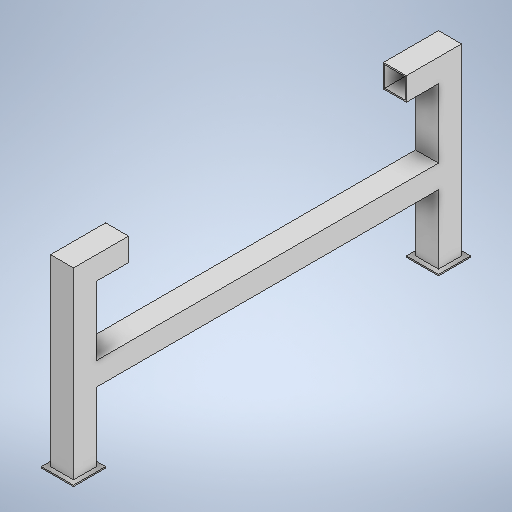
# Autodesk Inventor part: Soporte_altura
Saved by Autodesk Inventor 2025.2 (Build 292293000, 293)
## iProperties
Created: 2025-11-06
Part Number: Soporte_altura
Material: Genérico
Document SubType Name: Modeling
Designer: Dax
Density: 1 g/cm^3
Appearance: Valor por defecto
Author: Dax
Autodesk Inventor part; units mm, degrees
ref_plane "YZ Plane" through (0, 0, 0) normal (1, 0, 0) x (0, 1, 0)
ref_plane "XZ Plane" through (0, 0, 0) normal (0, 1, 0) x (-1, 0, 0)
ref_plane "XY Plane" through (0, 0, 0) normal (0, 0, 1) x (1, 0, 0)
sketch "Boceto1" plane through (0, 0, 0) normal (0, 0, 1) x (1, 0, 0)
  line L0 (-15.875, -15.875) -> (15.875, -15.875)
  line L1 (15.875, -15.875) -> (15.875, 15.875)
  line L2 (15.875, 15.875) -> (-15.875, 15.875)
  line L3 (-15.875, 15.875) -> (-15.875, -15.875)
  line L4 (-15.875, -15.875) -> (15.875, 15.875) construction
  line L5 (15.875, -15.875) -> (-15.875, 15.875) construction
  line L6 (-17.875, 17.875) -> (17.875, 17.875)
  line L7 (17.875, 17.875) -> (17.875, -17.875)
  line L8 (17.875, -17.875) -> (-17.875, -17.875)
  line L9 (-17.875, -17.875) -> (-17.875, 17.875)
  point P0 (0, 0)
  dimension "d0" = 31.75
  dimension "d1" = 31.75
  dimension "d2" = 2
  constraints: 20 end point, 4 parallel, 2 midpoint, 2 perpendicular, 1 horizontal, 3 other
  measures "d0" distance of L2.end L1.end
  measures "d1" distance of L1.end L0.end
  measures "d2" distance between parallel lines of L2 L6
extrude "Extrusión1" add sketch "Boceto1" along normal mid plane 604
sketch "Boceto2" plane through (-17.875, -17.875, 302) normal (0, -1, 0) x (1, 0, 0)
  line L0 (0, 0) -> (35.75, 0) projected
  line L1 (0, 0) -> (35.75, 0)
  line L2 (35.75, 0) -> (35.75, -35.75)
  line L3 (35.75, -35.75) -> (0, -35.75)
  line L4 (0, -35.75) -> (0, 0)
  line L5 (33.75, -33.75) -> (33.75, -2)
  line L6 (33.75, -2) -> (2, -2)
  line L7 (2, -2) -> (2, -33.75)
  line L8 (2, -33.75) -> (33.75, -33.75)
  line L9 (35.75, -604) -> (35.75, 0) projected
  line L10 (0, -604) -> (35.75, -604)
  line L11 (35.75, -604) -> (35.75, -568.25)
  line L12 (35.75, -568.25) -> (0, -568.25)
  line L13 (0, -568.25) -> (0, -604)
  line L14 (33.75, -570.25) -> (33.75, -602)
  line L15 (33.75, -602) -> (2, -602)
  line L16 (2, -602) -> (2, -570.25)
  line L17 (2, -570.25) -> (33.75, -570.25)
  point P0 (17.875, -302)
  dimension "d5" = 35.75
  dimension "d6" = 35.75
  dimension "d7" = 2
  constraints: 32 end point, 4 parallel, 2 perpendicular, 1 horizontal, 3 other
  measures "d5" distance of L2.end L3.end
  measures "d6" distance of L1.end L2.end
  measures "d7" distance between parallel lines of L2 L5
extrude "Extrusión2" add sketch "Boceto2" along normal blind 250 and the other way blind 35.75
sketch "Boceto3" plane through (-17.875, -17.875, -266.25) normal (0, 0, 1) x (1, 0, 0)
  line L0 (35.75, 35.75) -> (35.75, -250) projected
  line L1 (35.75, -107.125) -> (0, -107.125)
  line L2 (0, -107.125) -> (0, -142.875)
  line L3 (0, -142.875) -> (35.75, -142.875)
  line L4 (35.75, -142.875) -> (35.75, -107.125)
  line L5 (2, -109.125) -> (33.75, -109.125)
  line L6 (33.75, -109.125) -> (33.75, -140.875)
  line L7 (33.75, -140.875) -> (2, -140.875)
  line L8 (2, -140.875) -> (2, -109.125)
  point P0 (17.875, 17.875)
  point P1 (35.75, -142.875)
  dimension "d12" = 35.75
  dimension "d13" = 35.75
  dimension "d14" = 2
  constraints: 16 end point, 4 parallel, 2 perpendicular, 1 horizontal, 1 midpoint, 3 other
  measures "d12" distance of L3.end L2.end
  measures "d13" distance of L2.end L1.end
  measures "d14" distance between parallel lines of L1 L5
extrude "Extrusión3" add sketch "Boceto3" along normal blind 532.5
sketch "Boceto4" plane through (-17.875, 17.875, 302) normal (0, 1, 0) x (1, 0, 0)
  line L0 (0, 568.25) -> (35.75, 568.25) projected
  line L1 (35.75, 604) -> (35.75, 0) projected
  line L2 (35.75, 518.25) -> (0, 518.25)
  line L3 (0, 604) -> (0, 0) projected
  line L4 (17.875, 302) -> (67.1432, 302)
  line L5 (35.75, 85.75) -> (0, 85.75)
  line L6 (0, 518.25) -> (0, 85.75)
  line L7 (35.75, 85.75) -> (35.75, 518.25)
  dimension "d17" = 50
  constraints: 10 end point, 2 point on line, 2 symmetric about line, 1 collinear, 1 horizontal, 1 perpendicular
  measures "d17" distance of L0.end L2.start
extrude "Extrusión4" cut sketch "Boceto4" against normal blind 40 contours L2 L1 L5 L3
sketch "Boceto5" plane through (-17.875, -267.875, 302) normal (0, -1, 0) x (1, 0, 0)
  line L0 (33.75, -33.75) -> (33.75, -2) projected
  line L1 (33.75, -2) -> (2, -2) projected
  line L2 (-7.125, -42.875) -> (42.875, -42.875)
  line L3 (42.875, -42.875) -> (42.875, 7.125)
  line L4 (42.875, 7.125) -> (-7.125, 7.125)
  line L5 (-7.125, 7.125) -> (-7.125, -42.875)
  line L6 (-7.125, -42.875) -> (42.875, 7.125) construction
  line L7 (42.875, -42.875) -> (-7.125, 7.125) construction
  line L8 (-7.125, -561.125) -> (42.875, -561.125)
  line L9 (42.875, -561.125) -> (42.875, -611.125)
  line L10 (42.875, -611.125) -> (-7.125, -611.125)
  line L11 (-7.125, -611.125) -> (-7.125, -561.125)
  point P0 (17.875, -302)
  point P1 (17.875, -17.875)
  dimension "d20" = 50
  dimension "d21" = 50
  constraints: 20 end point, 2 midpoint, 2 parallel, 1 horizontal, 1 perpendicular
  measures "d20" distance of L4.end L3.end
  measures "d21" distance of L3.end L2.end
extrude "Extrusión5" add sketch "Boceto5" along normal blind 2
sketch "Boceto6" plane through (-15.875, -15.875, -266.25) normal (0, 0, 1) x (1, 0, 0)
  line L0 (0, 31.75) -> (31.75, 31.75) projected
  line L1 (31.75, 31.75) -> (31.75, 0) projected
  line L2 (0, 31.75) -> (31.75, 31.75)
  line L3 (31.75, 31.75) -> (31.75, 0)
  line L4 (31.75, 0) -> (0, 0)
  line L5 (0, 0) -> (0, 31.75)
  point P0 (15.875, 15.875)
  constraints: 8 end point, 2 parallel, 1 horizontal, 1 perpendicular
extrude "Extrusión6" cut sketch "Boceto6" along normal blind 550 and the other way blind 10
